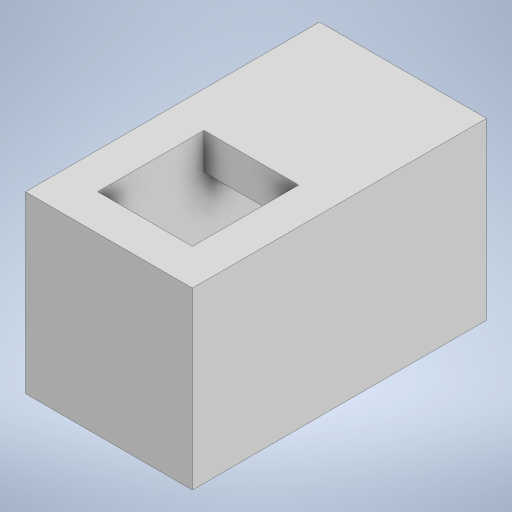
# Autodesk Inventor part: ADAPTER_AOM-brimrose-watercooled-cover-2
Saved by Autodesk Inventor 2024.2 (Build 282272000, 272)
## iProperties
Created: 2024-02-12
Part Number: ADAPTER_AOM-brimrose-watercooled-cover-2
Material: Generic
Document SubType Name: Modeling
Designer: fabig
Density: 1 g/cm^3
Appearance: Default
Author: fabig
Autodesk Inventor part; units mm, degrees
ref_plane "YZ Plane" through (0, 0, 0) normal (1, 0, 0) x (0, 1, 0)
ref_plane "XZ Plane" through (0, 0, 0) normal (0, 1, 0) x (-1, 0, 0)
ref_plane "XY Plane" through (0, 0, 0) normal (0, 0, 1) x (1, 0, 0)
sketch "Sketch1" plane through (0, 0, 0) normal (0, 1, 0) x (-1, 0, 0)
  point P0 (0, 0)
sketch "Sketch2" plane through (0, 0, 0) normal (0, 1, 0) x (-1, 0, 0)
  line L0 (-6.55, 15.35) -> (6.55, 15.35)
  line L1 (6.55, 15.35) -> (6.55, -15.35)
  line L2 (6.55, -15.35) -> (-6.55, -15.35)
  line L3 (-6.55, -15.35) -> (-6.55, 15.35)
  line L4 (-6.55, 15.35) -> (6.55, -15.35) construction
  line L5 (6.55, 15.35) -> (-6.55, -15.35) construction
  line L6 (-11.55, 20.35) -> (11.55, 20.35)
  line L7 (11.55, 20.35) -> (11.55, -20.35)
  line L8 (11.55, -20.35) -> (-11.55, -20.35)
  line L9 (-11.55, -20.35) -> (-11.55, 20.35)
  line L10 (-11.55, 20.35) -> (11.55, -20.35) construction
  line L11 (11.55, 20.35) -> (-11.55, -20.35) construction
  point P0 (0, 0)
  dimension "d0" = 13.1
  dimension "d1" = 30.7
  dimension "d2" = 23.1
  dimension "d3" = 40.7
  constraints: 24 end point, 4 midpoint, 4 parallel, 2 horizontal, 2 perpendicular
  measures "d0" distance of L1.end L2.end
  measures "d1" distance of L0.end L1.end
  measures "d2" distance of L7.end L8.end
  measures "d3" distance of L6.end L7.end
extrude "Extrusion1" add sketch "Sketch2" along normal blind 19.2
sketch "Sketch3" plane through (0, 19.2, 0) normal (0, 1, 0) x (1, 0, 0)
  line L0 (-11.55, -20.35) -> (11.55, -20.35)
  line L1 (11.55, -20.35) -> (11.55, 20.35)
  line L2 (11.55, 20.35) -> (-11.55, 20.35)
  line L3 (-11.55, 20.35) -> (-11.55, -20.35)
  point P0 (0, 0)
  constraints: 8 end point, 2 parallel, 1 horizontal, 1 perpendicular
extrude "Extrusion2" add sketch "Sketch3" along normal blind 5
sketch "Sketch4" plane through (0, 24.2, 0) normal (0, 1, 0) x (1, 0, 0)
  line L0 (-6.55, -15.35) -> (-6.55, 15.35) construction
  line L1 (6.55, -15.35) -> (-6.55, -15.35) construction
  line L2 (-6.55, -15.35) -> (-6.55, 15.35) construction
  line L3 (-6.55, 15.35) -> (6.55, 15.35) construction
  line L4 (6.55, 15.35) -> (6.55, -15.35) construction
  line L5 (6.55, -15.35) -> (-6.55, 15.35) construction
  line L6 (-6.55, -15.35) -> (6.55, 15.35) construction
  line L7 (6.55, 15.35) -> (6.55, -15.35) projected
  line L8 (-6.55, -15.35) -> (6.55, -15.35)
  line L9 (6.55, -15.35) -> (6.55, -0.65)
  line L10 (6.55, -0.65) -> (-6.55, -0.65)
  line L11 (-6.55, -0.65) -> (-6.55, -15.35)
  point P0 (0, 0)
  point P1 (6.55, -15.35)
  dimension "d8" = 14.7
  constraints: 20 end point, 4 parallel, 2 horizontal, 2 midpoint, 2 perpendicular, 1 point on line
  measures "d8" distance of L9.end L8.end
extrude "Extrusion3" cut sketch "Sketch4" against normal blind 5
body "Solid1"
